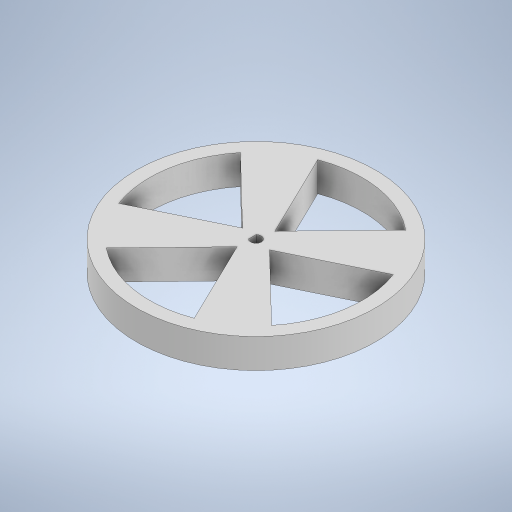
# Autodesk Inventor part: kolko1
Saved by Autodesk Inventor 2024.2 (Build 282272000, 272)
## iProperties
Created: 2024-05-09
Part Number: kolko1
Material: Ogólny
Document SubType Name: Modeling
Designer: rjane
Density: 1 g/cm^3
Appearance: Domyślna
Author: rjane
Autodesk Inventor part; units mm, degrees
ref_plane "YZ Plane" through (0, 0, 0) normal (1, 0, 0) x (0, 1, 0)
ref_plane "XZ Plane" through (0, 0, 0) normal (0, 1, 0) x (-1, 0, 0)
ref_plane "XY Plane" through (0, 0, 0) normal (0, 0, 1) x (1, 0, 0)
sketch "Szkic1" plane through (0, 0, 0) normal (0, 1, 0) x (-1, 0, 0)
  circle A0 centre (0, 0) radius 36.5
  circle A1 centre (0, 0) radius 32.5
  circle A2 centre (0, 0) radius 5
  circle A3 centre (0, 0) radius 1.65
  line L0 (1.15, 1.1832) -> (1.15, -1.1832)
  line L1 (-4.9328, 0.8172) -> (-25.2334, 20.4824)
  line L2 (-11.5454, 30.3802) -> (0.8172, 4.9328)
  line L3 (-4.9328, 0.8172) -> (-30.3802, -11.5454)
  line L4 (4.9328, -0.8172) -> (25.2334, -20.4824)
  line L5 (0.8172, 4.9328) -> (20.4824, 25.2334)
  line L6 (4.9328, -0.8172) -> (30.3802, 11.5454)
  line L7 (-0.8172, -4.9328) -> (-20.4824, -25.2334)
  line L8 (-0.8172, -4.9328) -> (11.5454, -30.3802)
  dimension "d1" = 65
  dimension "d0" = 73
  dimension "d2" = 10
  dimension "d3" = 3.3
  dimension "d4" = 2.8
  dimension "d6" = 20
  dimension "d7" = 20
  dimension "d14" = 20
  dimension "d15" = 20
  dimension "d16" = 5.75
  dimension "d17" = 5.75
  dimension "d18" = 5.75
  dimension "d19" = 5.75
  dimension "d20" = 70
  dimension "d21" = 70
  dimension "d22" = 70
  constraints: 18 end point, 6 point on circle, 4 coincident, 3 centre point, 1 vertical, 10 other
  measures "d0" diameter of A0
  measures "d2" diameter of A2
  measures "d3" diameter of A3
  measures "d6" angle of L2 L1
  measures "d7" angle of L6 L5
  measures "d14" angle of L4 L8
  measures "d15" angle of L7 L3
  measures "d16" vertical distance of L4.start L2.end
  measures "d17" vertical distance of L7.start L1.start
  measures "d18" horizontal distance of L7.start L4.start
  measures "d19" horizontal distance of L2.end L1.start
  measures "d20" angle of L3 L1
  measures "d21" angle of L5 L2
  measures "d22" angle of L4 L6
extrude "Wyciągnięcie proste1" add sketch "Szkic1" along normal blind 9 contours A0 | L6 A2 L5 A1 | A1 L8 A2 L4 | A2 | L2 A2 L1 A1 | L7 A1 L3 A2 | A3 L0 picked at (1.3167, 0)
